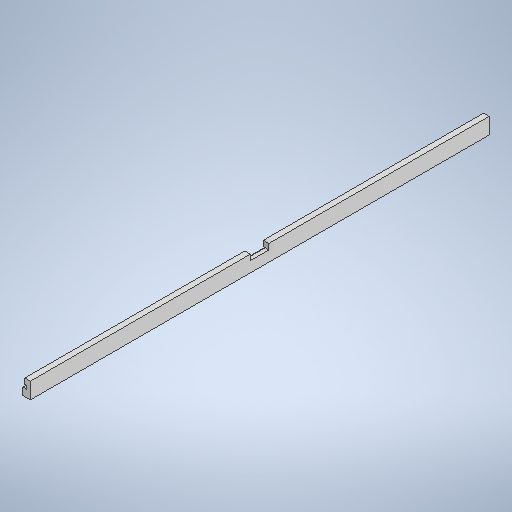
# Autodesk Inventor part: Top Case Rail
Saved by Autodesk Inventor 2025 (Build 290162000, 162)
## iProperties
Created: 2024-07-16
Part Number: Top Case Rail
Material: Generic
Document SubType Name: Modeling
Designer: adam
Density: 1 g/cm^3
Appearance: Default
Author: adam
Autodesk Inventor part; units mm, degrees
ref_plane "YZ Plane" through (0, 0, 0) normal (1, 0, 0) x (0, 1, 0)
ref_plane "XZ Plane" through (0, 0, 0) normal (0, 1, 0) x (-1, 0, 0)
ref_plane "XY Plane" through (0, 0, 0) normal (0, 0, 1) x (1, 0, 0)
sketch "Sketch1" plane through (0, 0, 0) normal (0, 0, 1) x (1, 0, 0)
  line L0 (0, 4.75) -> (2, 4.75)
  line L1 (2, 4.75) -> (2, -4)
  line L2 (2, -4) -> (0, -4)
  line L3 (0, -4) -> (0, 4.75) construction
  line L4 (0, -4) -> (-2, -4)
  line L5 (-2, -4) -> (-2, 0)
  line L6 (-2, 0) -> (0, 0)
  line L7 (0, 4.75) -> (-1, 4.75)
  line L8 (-1, 4.75) -> (-1, 1.75)
  line L9 (-1, 1.75) -> (0, 1.75)
  line L10 (0, 1.75) -> (0, 4.75) construction
  line L11 (0, 1.75) -> (0, 0)
  point P0 (0, 0)
  point P1 (0, 0.375)
  point P2 (1, 4.75)
  dimension "d0" = 4
  dimension "d1" = 2
  dimension "d5" = 2
  dimension "d6" = 1.75
  dimension "d7" = 4
  dimension "d11" = 3
  dimension "d12" = 3
  constraints: 24 end point, 5 parallel, 3 horizontal, 3 perpendicular, 2 midpoint, 1 collinear, 1 point on line
  measures "d0" distance from line of L2 point (0, 0)
  measures "d1" distance from line of L1 point (0, 0.375)
  measures "d5" distance between parallel lines of L3 L5
  measures "d6" distance between parallel lines of L6 L9
  measures "d7" distance of L4.end L5.end
  measures "d11" distance between parallel lines of L0 L9
  measures "d12" distance between parallel lines of L1 L8
extrude "Extrusion1" add sketch "Sketch1" along normal blind 248
sketch "Sketch2" plane through (-1, 4.75, 248) normal (0, 1, 0) x (1, 0, 0)
  line L0 (3, 248) -> (3, 0) construction
  line L1 (3, 124) -> (1, 124) construction
  line L2 (1, 248) -> (1, 0) construction
  line L3 (3, 129) -> (1, 129)
  line L4 (1, 129) -> (1, 119) construction
  line L5 (1, 119) -> (3, 119) construction
  line L6 (3, 119) -> (3, 129)
  line L7 (3, 124) -> (1, 124) construction
  line L8 (3, 119) -> (1, 119)
  line L9 (1, 129) -> (0, 129)
  line L10 (0, 248) -> (0, 0) projected
  line L11 (0, 129) -> (0, 119)
  line L12 (0, 119) -> (1, 119)
  dimension "d13" = 10
  constraints: 20 end point, 4 midpoint, 3 perpendicular, 3 point on line, 2 horizontal, 2 parallel, 1 collinear, 1 vertical
  measures "d13" distance of L4.end L3.end
extrude "Extrusion2" cut sketch "Sketch2" against normal up to surface (3 mm away)
body "Solid1"
